mine3 (Autodesk Fusion 360 design; units mm, degrees)
Autodesk Fusion 360 part; units mm, degrees
note: some values were not read from the file. Set by a fixed rule: which sketch regions a step uses.
sketch "Sketch3" plane through (0, 0, 0) normal (1, 0, 0) x (0, 1, 0)
  line L0 (-6.4831, 19) -> (6.5169, 19)
  line L1 (6.5169, 19) -> (6.5169, 17.6307)
  line L2 (6.5169, 17.6307) -> (-6.4831, 17.6307)
  line L3 (-6.4831, 17.6307) -> (-6.4831, 19)
  line L4 (-10.0331, 0) -> (9.9669, 0)
  line L5 (9.9669, 0) -> (9.9669, 3.9074)
  line L6 (9.9669, 3.9074) -> (-10.0331, 3.9074)
  line L7 (-10.0331, 3.9074) -> (-10.0331, 0)
  dimension "d21" = 13
  dimension "d22" = 20
  constraint horizontal L0
  constraint vertical L1
  constraint horizontal L2
  constraint vertical L3
  constraint horizontal L4
  constraint vertical L5
  constraint horizontal L6
  constraint vertical L7
  measures "d21" distance of L1.end L2.end
  measures "d22" distance of L5.end L6.end
sketch "Sketch1" plane through (0, 0, 0) normal (1, 0, 0) x (0, 1, 0)
  line L0 (0, 0) -> (10, 0)
  line L1 (0, 0) -> (23.5, 0)
  line L2 (0, 163.4986) -> (19.1386, -149.4155) construction
  line L3 (0, 0) -> (0, -100)
  line L4 (0, -100) -> (16.1163, -100)
  line L5 (23.5, 0) -> (23.5, 26.5)
  line L6 (23.5, 26.5) -> (26, 26.5)
  line L7 (26, 0) -> (26, 26.5)
  line L8 (23.5, 21.5919) -> (12, 21.5919)
  line L9 (10, 0) -> (23.5, 0)
  line L10 (10, 0) -> (16.1163, -100)
  line L11 (26, 0) -> (26, -2.5)
  line L12 (26, -2.5) -> (12.6576, -2.5)
  line L13 (12.6576, -2.5) -> (18.6209, -100)
  line L14 (16.1163, -100) -> (18.6209, -100)
  line L15 (10, 0) -> (23.5, 0) construction
  line L16 (26, 0) -> (155, 0) construction
  dimension "d1" = 10
  dimension "d2" = 23.5
  dimension "d5" = 100
  dimension "d6" = 26.5
  dimension "d7" = 2.5
  dimension "d8" = 2.5
  dimension "d11" = 3.5
  dimension "d20" = 16.1163
  dimension "d23" = 2.5
  constraint coincident L0.start L1.start
  constraint horizontal L0
  constraint parallel L0 L1
  constraint horizontal L15
  constraint perpendicular L1 L3
  constraint coincident L2 L4.end
  constraint perpendicular L3 L4
  constraint perpendicular L1 L5
  constraint perpendicular L5 L6
  constraint coincident L5 L8.start
  constraint perpendicular L5 L8
  constraint coincident L0.end L2
  constraint perpendicular L11 L15
  constraint perpendicular L11 L12
  constraint horizontal L14
  constraint collinear L15 L16
  measures "d1" distance of L0.start L0.end
  measures "d2" distance of L0.start L1.end
  measures "d5" distance of L0.start L3.end
  measures "d6" distance of L1.end L5.end
  measures "d7" distance of L5.end L6.end
  measures "d8" distance of L1.end L7.start
  measures "d11" angle of L2 L3
  measures "d20" distance of L3.end L4.end
  measures "d23" distance of L7.start L11.end
revolve "Revolve1" add sketch "Sketch1" angle 360 about axis through (0, 0, 0) along (0, 0, -1) contours L1 L5 L6 L7 L9 L10 L11 L12 L13 L14
ref_plane "WorkPlane1" through (0, 23.5, 20.2419) normal (0, -1, 0) x (1, 0, 0)
sketch "Sketch2" plane through (0, 23.5, 20.3906) normal (0, -1, 0) x (1, 0, 0)
  circle A0 centre (0, 1.2013) radius 3
  point P0 (0, 1.2013)
  dimension "d13" = 6
  constraint coincident P0 A0.centre
  measures "d13" diameter of A0
extrude "Extrude1" cut sketch "Sketch2" along normal mid plane 42
pattern_circular "C-Pattern1" count 3 over 360 about axis through (0, 0, 1.75) along (0, 0, 1) of "Extrude1"
chamfer "Chamfer1" distance 1 distance2 2 1 edges at (-21.9097, 8.498, 26.5) measured on face at (-1.2917, 25.0699, 26.5)
fillet "Fillet1" radius 45 1 edges at (-11.801, 4.5772, -2.5)
